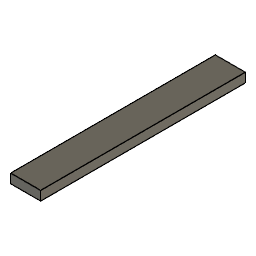
Canal - blocker v2 (Autodesk Fusion 360 design; units mm, degrees)
Autodesk Fusion 360 part; units mm, degrees
sketch "Sketch1" plane through (0, 0, 0) normal (0, 1, 0) x (1, 0, 0)
  line L0 (10, -10) -> (12.9, -10)
  line L1 (12.9, -10) -> (12.9, -9.1)
  line L2 (12.9, -9.1) -> (10, -9.1)
  line L3 (10, -9.1) -> (10, -10)
  dimension "d1" = 2.9
  dimension "d2" = 0.9
  constraint horizontal L0
  constraint vertical L1
  constraint horizontal L2
  constraint vertical L3
  measures "d1" distance of L0.start L0.end
  measures "d2" distance of L0.start L2.end
extrude "Extrude1" add sketch "Sketch1" along normal blind 19.75
